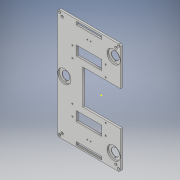
# Autodesk Inventor part: Grundplatte
Saved by Autodesk Inventor 2017 (Build 210142000, 142)
## iProperties
Part Number: Grundplatte
Material: Generisch
Document SubType Name: Modeling
Designer: Dima
Density: 1 g/cm^3
Appearance: Vorgabe
Author: Dima
Autodesk Inventor part; units mm, degrees
ref_plane "YZ Plane" through (0, 0, 0) normal (1, 0, 0) x (0, 1, 0)
ref_plane "XZ Plane" through (0, 0, 0) normal (0, 1, 0) x (-1, 0, 0)
ref_plane "XY Plane" through (0, 0, 0) normal (0, 0, 1) x (1, 0, 0)
sketch "Skizze1" plane through (0, 0, 0) normal (0, 1, 0) x (-1, 0, 0)
  line L0 (132.5635, 175.274) -> (-67.4365, 175.274)
  line L1 (-67.4365, 175.274) -> (-67.4365, -174.726)
  line L2 (-67.4365, -174.726) -> (132.5635, -174.726)
  line L3 (132.5635, -174.726) -> (132.5635, 175.274)
  line L4 (354.7243, 0.274) -> (-224.9528, 0.274)
  point P0 (0, 0)
  dimension "d0" = 350
  dimension "d1" = 200
  dimension "d2" = 175
  dimension "d3" = 175
  constraints: 10 end point, 2 horizontal, 2 parallel, 1 perpendicular
  measures "d0" distance of L2.end L0.start
  measures "d1" distance of L0.start L0.end
  measures "d2" distance between parallel lines of L0 L4
  measures "d3" distance between parallel lines of L2 L4
extrude "Extrusion1" add sketch "Skizze1" along normal blind 6
chamfer "Fase1" distance 5 angle 45 1 edges at (-132.5635, 3, 175.274)
chamfer "Fase2" distance 5 angle 45 1 edges at (67.4365, 3, 175.274)
chamfer "Fase3" distance 5 angle 45 1 edges at (67.4365, 3, -174.726)
chamfer "Fase4" distance 5 angle 45 1 edges at (-132.5635, 3, -174.726)
sketch "Skizze3" plane through (0, 6, 0) normal (0, 1, 0) x (1, 0, 0)
  point P0 (0, 0)
sketch "Skizze4" plane through (0, 6, 0) normal (0, 1, 0) x (1, 0, 0)
  point P0 (0, 0)
sketch "Skizze5" plane through (0, 6, 0) normal (0, 1, 0) x (1, 0, 0)
  line L0 (140.4629, -0.274) -> (-239.786, -0.274)
  line L1 (-32.5635, -205.6988) -> (-32.5635, 212.7513)
  line L2 (-127.5635, -175.274) -> (62.4365, -175.274) projected
  line L3 (62.4365, 174.726) -> (-127.5635, 174.726) projected
  line L4 (67.4365, -170.274) -> (67.4365, 169.726) projected
  line L5 (-132.5635, 169.726) -> (-132.5635, -170.274) projected
  line L6 (67.4365, -55.274) -> (-52.5635, -55.274)
  line L7 (-52.5635, -55.274) -> (-52.5635, 54.726)
  line L8 (-52.5635, 54.726) -> (67.4365, 54.726)
  line L9 (67.4365, 54.726) -> (67.4365, -55.274)
  point P0 (0, 0)
  dimension "d18" = 175
  dimension "d19" = 175
  dimension "d20" = 100
  dimension "d21" = 100
  dimension "d22" = 120
  dimension "d23" = 120
  dimension "d24" = 80
  dimension "d62" = 110
  constraints: 12 end point, 2 horizontal, 2 parallel, 1 perpendicular, 1 point on line, 1 vertical
  measures "d18" distance between parallel lines of L2 L0
  measures "d19" distance between parallel lines of L3 L0
  measures "d20" distance between parallel lines of L4 L1
  measures "d21" distance between parallel lines of L1 L5
  measures "d22" distance between parallel lines of L3 L8
  measures "d23" distance between parallel lines of L6 L2
  measures "d24" distance between parallel lines of L5 L7
  measures "d62" distance between parallel lines of L8 L6
extrude "Extrusion2" cut sketch "Skizze5" against normal blind 6
sketch "Skizze10" plane through (0, 6, 0) normal (0, 1, 0) x (1, 0, 0)
  line L0 (7.4365, -170.274) -> (-72.5635, -170.274)
  line L1 (-72.5635, -170.274) -> (-72.5635, -160.274)
  line L2 (-72.5635, -160.274) -> (7.4365, -160.274)
  line L3 (7.4365, -160.274) -> (7.4365, -170.274)
  line L4 (7.4365, 74.726) -> (-72.5635, 74.726)
  line L5 (-72.5635, 74.726) -> (-72.5635, 104.726)
  line L6 (-72.5635, 104.726) -> (7.4365, 104.726)
  line L7 (7.4365, 104.726) -> (7.4365, 74.726)
  line L8 (7.4365, 159.726) -> (-72.5635, 159.726)
  line L9 (-72.5635, 159.726) -> (-72.5635, 169.726)
  line L10 (-72.5635, 169.726) -> (7.4365, 169.726)
  line L11 (7.4365, 169.726) -> (7.4365, 159.726)
  line L12 (-52.5635, 54.726) -> (67.4365, 54.726) construction
  line L13 (67.4365, 54.726) -> (67.4365, 169.726) construction
  line L14 (62.4365, 174.726) -> (67.4365, 169.726) construction
  line L15 (62.4365, 174.726) -> (-127.5635, 174.726) construction
  line L16 (-132.5635, 169.726) -> (-127.5635, 174.726) construction
  line L17 (-132.5635, 169.726) -> (-132.5635, -170.274) construction
  line L18 (-127.5635, -175.274) -> (-132.5635, -170.274) construction
  line L19 (-127.5635, -175.274) -> (62.4365, -175.274) construction
  line L20 (67.4365, -170.274) -> (62.4365, -175.274) construction
  line L21 (67.4365, -170.274) -> (67.4365, -55.274) construction
  line L22 (67.4365, -55.274) -> (-52.5635, -55.274) construction
  line L23 (-52.5635, -55.274) -> (-52.5635, 54.726) construction
  line L24 (-127.5635, -175.274) -> (62.4365, -175.274) projected
  line L25 (7.4365, -105.274) -> (-72.5635, -105.274)
  line L26 (-72.5635, -105.274) -> (-72.5635, -75.274)
  line L27 (-72.5635, -75.274) -> (7.4365, -75.274)
  line L28 (7.4365, -75.274) -> (7.4365, -105.274)
  point P0 (0, 0)
  point P1 (-32.5635, -175.274)
  point P2 (-32.5635, -170.274)
  point P3 (-32.5635, -160.274)
  point P4 (-32.5635, 74.726)
  point P5 (-32.5635, -175.274)
  point P6 (-32.5635, 104.726)
  point P7 (-32.5635, 159.726)
  point P8 (-32.5635, -105.274)
  dimension "d99" = 5
  dimension "d100" = 10
  dimension "d101" = 10
  dimension "d102" = 5
  dimension "d106" = 55
  dimension "d107" = 55
  dimension "d108" = 30
  dimension "d109" = 30
  dimension "d110" = 80
  dimension "d111" = 80
  constraints: 32 end point, 8 midpoint, 8 parallel, 6 vertical alignment, 4 horizontal, 4 perpendicular
  measures "d99" distance between parallel lines of L0 L19
  measures "d100" distance between parallel lines of L2 L0
  measures "d101" distance between parallel lines of L10 L8
  measures "d102" distance between parallel lines of L15 L10
  measures "d106" distance between parallel lines of L2 L25
  measures "d107" distance between parallel lines of L8 L6
  measures "d108" distance between parallel lines of L25 L27
  measures "d109" distance of L4.end L5.end
  measures "d110" distance of L25.start L25.end
  measures "d111" distance of L0.start L0.end
extrude "Extrusion4" cut sketch "Skizze10" against normal through all
sketch "Skizze11" plane through (0, 0, 0) normal (0, -1, 0) x (1, 0, 0)
  line L0 (7.4365, -74.726) -> (7.4365, -104.726) construction
  line L1 (7.4365, -104.726) -> (-72.5635, -104.726) construction
  line L2 (-72.5635, -104.726) -> (-72.5635, -74.726) construction
  line L3 (-72.5635, -74.726) -> (7.4365, -74.726) construction
  line L4 (7.4365, 170.274) -> (7.4365, 160.274) construction
  line L5 (7.4365, 160.274) -> (-72.5635, 160.274) construction
  line L6 (-72.5635, 160.274) -> (-72.5635, 170.274) construction
  line L7 (-72.5635, 170.274) -> (7.4365, 170.274) construction
  line L8 (7.4365, -159.726) -> (7.4365, -169.726) construction
  line L9 (7.4365, -169.726) -> (-72.5635, -169.726) construction
  line L10 (-72.5635, -169.726) -> (-72.5635, -159.726) construction
  line L11 (-72.5635, -159.726) -> (7.4365, -159.726) construction
  line L12 (7.4365, 105.274) -> (7.4365, 75.274) construction
  line L13 (7.4365, 75.274) -> (-72.5635, 75.274) construction
  line L14 (-72.5635, 75.274) -> (-72.5635, 105.274) construction
  line L15 (-72.5635, 105.274) -> (7.4365, 105.274) construction
  line L16 (67.4365, -54.726) -> (-52.5635, -54.726) construction
  line L17 (-52.5635, -54.726) -> (-52.5635, 55.274) construction
  line L18 (-52.5635, 55.274) -> (67.4365, 55.274) construction
  line L19 (67.4365, 170.274) -> (67.4365, 55.274) construction
  line L20 (62.4365, 175.274) -> (67.4365, 170.274) construction
  line L21 (-127.5635, 175.274) -> (62.4365, 175.274) construction
  line L22 (-132.5635, 170.274) -> (-127.5635, 175.274) construction
  line L23 (-132.5635, -169.726) -> (-132.5635, 170.274) construction
  line L24 (-127.5635, -174.726) -> (-132.5635, -169.726) construction
  line L25 (62.4365, -174.726) -> (-127.5635, -174.726) construction
  line L26 (67.4365, -169.726) -> (62.4365, -174.726) construction
  line L27 (67.4365, -54.726) -> (67.4365, -169.726) construction
  circle A0 centre (-110.5635, 0.274) radius 21
  circle A1 centre (45.4365, 132.274) radius 21
  circle A2 centre (45.4365, -131.726) radius 21
  line L28 (-131.5635, -14.726) -> (-131.5635, 15.274) construction
  line L29 (-132.5635, -169.726) -> (-132.5635, 170.274) construction
  line L30 (66.4365, 132.274) -> (66.4365, 153.274) construction
  line L31 (66.4365, 153.274) -> (45.4365, 153.274) construction
  line L32 (45.4365, -152.726) -> (66.4365, -152.726) construction
  line L33 (66.4365, -152.726) -> (66.4365, -131.726) construction
  point P0 (0, 0)
  point P1 (-132.5635, 0.274)
  point P2 (-131.5635, 0.274)
  point P3 (-132.5635, 0.274)
  dimension "d114" = 42
  dimension "d115" = 42
  dimension "d116" = 42
  dimension "d117" = 30
  dimension "d118" = 1
  dimension "d119" = 1
  dimension "d120" = 22
  dimension "d121" = 22
  constraints: 10 end point, 5 tangent, 4 horizontal alignment, 3 centre point, 3 midpoint, 3 vertical alignment, 2 horizontal, 2 vertical, 1 perpendicular
  measures "d114" diameter of A0
  measures "d115" diameter of A1
  measures "d116" diameter of A2
  measures "d117" distance of L28.start L28.end
  measures "d118" distance between parallel lines of L23 L28
  measures "d119" distance between parallel lines of L19 L30
  measures "d120" distance between parallel lines of L25 L32
  measures "d121" distance between parallel lines of L21 L31
extrude "Extrusion5" cut sketch "Skizze11" against normal blind 5
sketch "Skizze12" plane through (45.4365, 5, -131.726) normal (0, -1, 0) x (1, 0, 0)
  circle A0 centre (0, 0) radius 21 projected
  circle A1 centre (-156, 132) radius 21 projected
  circle A2 centre (0, 264) radius 21 projected
  circle A3 centre (0, 264) radius 21 projected
  point P0 (-45.4365, 131.726)
  constraints: 3 coincident
hole "Bohrung1" at (-110.5635, 5, 0.274) at (45.4365, 5, 132.274) at (45.4365, 5, -131.726) direction (0, 1, 0) diameter 25 end through all
sketch "Skizze13" plane through (0, 0, 0) normal (0, -1, 0) x (1, 0, 0)
  circle A0 centre (45.4365, 132.274) radius 21 construction
  circle A1 centre (-110.5635, 0.274) radius 21 construction
  circle A2 centre (45.4365, -131.726) radius 21 construction
  line L0 (7.4365, -74.726) -> (7.4365, -104.726) construction
  line L1 (7.4365, -104.726) -> (-72.5635, -104.726) construction
  line L2 (-72.5635, -104.726) -> (-72.5635, -74.726) construction
  line L3 (-72.5635, -74.726) -> (7.4365, -74.726) construction
  line L4 (7.4365, 170.274) -> (7.4365, 160.274) construction
  line L5 (7.4365, 160.274) -> (-72.5635, 160.274) construction
  line L6 (-72.5635, 160.274) -> (-72.5635, 170.274) construction
  line L7 (-72.5635, 170.274) -> (7.4365, 170.274) construction
  line L8 (7.4365, -159.726) -> (7.4365, -169.726) construction
  line L9 (7.4365, -169.726) -> (-72.5635, -169.726) construction
  line L10 (-72.5635, -169.726) -> (-72.5635, -159.726) construction
  line L11 (-72.5635, -159.726) -> (7.4365, -159.726) construction
  line L12 (7.4365, 105.274) -> (7.4365, 75.274) construction
  line L13 (7.4365, 75.274) -> (-72.5635, 75.274) construction
  line L14 (-72.5635, 75.274) -> (-72.5635, 105.274) construction
  line L15 (-72.5635, 105.274) -> (7.4365, 105.274) construction
  line L16 (67.4365, -54.726) -> (-52.5635, -54.726) construction
  line L17 (-52.5635, -54.726) -> (-52.5635, 55.274) construction
  line L18 (-52.5635, 55.274) -> (67.4365, 55.274) construction
  line L19 (67.4365, 170.274) -> (67.4365, 55.274) construction
  line L20 (62.4365, 175.274) -> (67.4365, 170.274) construction
  line L21 (-127.5635, 175.274) -> (62.4365, 175.274) construction
  line L22 (-132.5635, 170.274) -> (-127.5635, 175.274) construction
  line L23 (-132.5635, -169.726) -> (-132.5635, 170.274) construction
  line L24 (-127.5635, -174.726) -> (-132.5635, -169.726) construction
  line L25 (62.4365, -174.726) -> (-127.5635, -174.726) construction
  line L26 (67.4365, -169.726) -> (62.4365, -174.726) construction
  line L27 (67.4365, -54.726) -> (67.4365, -169.726) construction
  point P0 (0, 0)
  point P1 (-125.5635, -167.726)
  point P2 (-117.5635, -159.726)
  point P3 (-125.5635, 168.274)
  point P4 (-117.5635, 160.274)
  point P5 (52.4365, 160.274)
  point P6 (60.4365, 168.274)
  point P7 (60.4365, -167.726)
  point P8 (52.4365, -159.726)
  dimension "d131" = 7
  dimension "d132" = 7
  dimension "d133" = 15
  dimension "d134" = 15
  dimension "d135" = 7
  dimension "d136" = 7
  dimension "d137" = 7
  dimension "d138" = 7
  dimension "d139" = 7
  dimension "d140" = 7
  dimension "d141" = 15
  dimension "d142" = 15
  dimension "d143" = 15
  dimension "d144" = 15
  dimension "d145" = 15
  dimension "d146" = 15
  measures "d131" distance from line of point (-125.564, -167.726) L25
  measures "d132" distance from line of L23 point (-125.564, -167.726)
  measures "d133" distance from line of L25 point (-117.564, -159.726)
  measures "d134" distance from line of L23 point (-117.564, -159.726)
  measures "d135" distance from line of L21 point (-125.564, 168.274)
  measures "d136" distance from line of L23 point (-125.564, 168.274)
  measures "d137" distance from line of L21 point (60.436, 168.274)
  measures "d138" distance from line of L19 point (60.436, 168.274)
  measures "d139" distance from line of L27 point (60.436, -167.726)
  measures "d140" distance from line of L25 point (60.436, -167.726)
  measures "d141" distance from line of L21 point (-117.564, 160.274)
  measures "d142" distance from line of L23 point (-117.564, 160.274)
  measures "d143" distance from line of L19 point (52.436, 160.274)
  measures "d144" distance from line of L21 point (52.436, 160.274)
  measures "d145" distance from line of L27 point (52.436, -159.726)
  measures "d146" distance from line of L25 point (52.436, -159.726)
hole "Bohrung2" at (60.4365, 0, -167.726) at (52.4365, 0, -159.726) at (-117.5635, 0, -159.726) at (-125.5635, 0, -167.726) at (-117.5635, 0, 160.274) at (-125.5635, 0, 168.274) at (52.4365, 0, 160.274) at (60.4365, 0, 168.274) direction (0, 1, 0) diameter 4.5 end through all counterbore diameter 8 counterbore depth 4
sketch "Skizze14" plane through (0, 0, 0) normal (0, -1, 0) x (1, 0, 0)
  circle A0 centre (52.4365, 160.274) radius 4 construction
  circle A1 centre (-117.5635, 160.274) radius 4 construction
  circle A2 centre (-117.5635, -159.726) radius 4 construction
  circle A3 centre (60.4365, -167.726) radius 4 construction
  circle A4 centre (52.4365, -159.726) radius 4 construction
  circle A5 centre (-125.5635, -167.726) radius 4 construction
  circle A6 centre (-125.5635, 168.274) radius 4 construction
  circle A7 centre (60.4365, 168.274) radius 4 construction
  circle A8 centre (45.4365, 132.274) radius 21 construction
  circle A9 centre (-110.5635, 0.274) radius 21 construction
  circle A10 centre (45.4365, -131.726) radius 21 construction
  line L0 (7.4365, -74.726) -> (7.4365, -104.726) construction
  line L1 (7.4365, -104.726) -> (-72.5635, -104.726) construction
  line L2 (-72.5635, -104.726) -> (-72.5635, -74.726) construction
  line L3 (-72.5635, -74.726) -> (7.4365, -74.726) construction
  line L4 (7.4365, 170.274) -> (7.4365, 160.274) construction
  line L5 (7.4365, 160.274) -> (-72.5635, 160.274) construction
  line L6 (-72.5635, 160.274) -> (-72.5635, 170.274) construction
  line L7 (-72.5635, 170.274) -> (7.4365, 170.274) construction
  line L8 (7.4365, -159.726) -> (7.4365, -169.726) construction
  line L9 (7.4365, -169.726) -> (-72.5635, -169.726) construction
  line L10 (-72.5635, -169.726) -> (-72.5635, -159.726) construction
  line L11 (-72.5635, -159.726) -> (7.4365, -159.726) construction
  line L12 (7.4365, 105.274) -> (7.4365, 75.274) construction
  line L13 (7.4365, 75.274) -> (-72.5635, 75.274) construction
  line L14 (-72.5635, 75.274) -> (-72.5635, 105.274) construction
  line L15 (-72.5635, 105.274) -> (7.4365, 105.274) construction
  line L16 (67.4365, -54.726) -> (-52.5635, -54.726) construction
  line L17 (-52.5635, -54.726) -> (-52.5635, 55.274) construction
  line L18 (-52.5635, 55.274) -> (67.4365, 55.274) construction
  line L19 (67.4365, 170.274) -> (67.4365, 55.274) construction
  line L20 (62.4365, 175.274) -> (67.4365, 170.274) construction
  line L21 (-127.5635, 175.274) -> (62.4365, 175.274) construction
  line L22 (-132.5635, 170.274) -> (-127.5635, 175.274) construction
  line L23 (-132.5635, -169.726) -> (-132.5635, 170.274) construction
  line L24 (-127.5635, -174.726) -> (-132.5635, -169.726) construction
  line L25 (62.4365, -174.726) -> (-127.5635, -174.726) construction
  line L26 (67.4365, -169.726) -> (62.4365, -174.726) construction
  line L27 (67.4365, -54.726) -> (67.4365, -169.726) construction
  line L28 (-32.5635, 105.274) -> (-32.5635, 75.274) construction
  point P0 (0, 0)
  point P1 (-85.0635, -97.226)
  point P2 (-85.0635, -62.226)
  point P3 (19.9365, -97.226)
  point P4 (19.9365, -62.226)
  point P5 (-85.0635, 62.774)
  point P6 (-85.0635, 97.774)
  point P7 (19.9365, 62.774)
  point P8 (19.9365, 97.774)
  dimension "d154" = 105
  dimension "d155" = 35
  dimension "d156" = 35
  dimension "d157" = 7.5
  dimension "d158" = 7.5
  constraints: 6 vertical alignment, 4 horizontal alignment, 2 end point, 2 midpoint, 1 symmetric about line
  measures "d154" distance of point (19.936, 97.774) point (-85.064, 97.774)
  measures "d155" distance of point (-85.064, 62.774) point (-85.064, 97.774)
  measures "d156" distance of point (-85.064, -97.226) point (-85.064, -62.226)
  measures "d157" distance from line of L18 point (19.936, 62.774)
  measures "d158" distance from line of L16 point (19.936, -62.226)
hole "Bohrung3" at (-85.0635, 0, -97.226) at (-85.0635, 0, -62.226) at (19.9365, 0, -97.226) at (19.9365, 0, -62.226) at (19.9365, 0, 62.774) at (19.9365, 0, 97.774) at (-85.0635, 0, 62.774) at (-85.0635, 0, 97.774) direction (0, 1, 0) diameter 4.134 depth 14.2 tip angle 118 thread size "M5x0.8" class "6H" standard "ISO Metric profile"
sketch "Skizze15" plane through (45.4365, 5, -131.726) normal (0, -1, 0) x (1, 0, 0)
  circle A0 centre (0, 264) radius 12.5 construction
  circle A1 centre (0, 0) radius 21 construction
  circle A2 centre (0, 0) radius 12.5 construction
  circle A3 centre (-156, 132) radius 21 construction
  circle A4 centre (-156, 132) radius 12.5 construction
  circle A5 centre (0, 264) radius 21 construction
  line L0 (0, -21) -> (0, 21) construction
  line L1 (-156, 111) -> (-156, 153) construction
  line L2 (0, 243) -> (0, 285) construction
  line L3 (-21, 264) -> (21, 264) construction
  line L4 (-177, 132) -> (-135, 132) construction
  line L5 (-178, -38) -> (-178, 302) construction
  line L6 (-21, 0) -> (21, 0) construction
  line L7 (22, 77) -> (22, -38) construction
  point P0 (-45.4365, 131.726)
  point P1 (0, 15)
  point P2 (0, -15)
  point P3 (-156, 117)
  point P4 (-156, 147)
  point P5 (0, 249)
  point P6 (0, 279)
  point P7 (0, 0)
  point P8 (0, 264)
  point P9 (-156, 132)
  dimension "d166" = 30
  dimension "d167" = 30
  dimension "d168" = 30
  constraints: 12 end point, 12 point on circle, 9 midpoint, 8 point on line, 3 symmetric about line, 2 perpendicular, 1 horizontal, 1 parallel, 1 vertical
  measures "d166" distance of point (-156, 147) point (-156, 117)
  measures "d167" distance of point (0, 15) point (0, -15)
  measures "d168" distance of point (0, 279) point (0, 249)
hole "Bohrung4" at (45.4365, 5, -146.726) at (45.4365, 5, -116.726) at (-110.5635, 5, -14.726) at (-110.5635, 5, 15.274) at (45.4365, 5, 117.274) at (45.4365, 5, 147.274) direction (0, 1, 0) diameter 2.459 depth 8.8 tip angle 118 thread size "M3x0.5" class "6H" standard "ISO Metric profile"
sketch "Skizze16" plane through (0, 0, 0) normal (0, -1, 0) x (1, 0, 0)
  circle A0 centre (-85.0635, 62.774) radius 2.067 construction
  circle A1 centre (19.9365, 62.774) radius 2.067 construction
  circle A2 centre (19.9365, -97.226) radius 2.067 construction
  circle A3 centre (-85.0635, -97.226) radius 2.067 construction
  circle A4 centre (-85.0635, -62.226) radius 2.067 construction
  circle A5 centre (19.9365, -62.226) radius 2.067 construction
  circle A6 centre (19.9365, 97.774) radius 2.067 construction
  circle A7 centre (-85.0635, 97.774) radius 2.067 construction
  circle A8 centre (52.4365, 160.274) radius 4 construction
  circle A9 centre (-117.5635, 160.274) radius 4 construction
  circle A10 centre (-117.5635, -159.726) radius 4 construction
  circle A11 centre (60.4365, -167.726) radius 4 construction
  circle A12 centre (52.4365, -159.726) radius 4 construction
  circle A13 centre (-125.5635, -167.726) radius 4 construction
  circle A14 centre (-125.5635, 168.274) radius 4 construction
  circle A15 centre (60.4365, 168.274) radius 4 construction
  circle A16 centre (45.4365, 132.274) radius 21 construction
  circle A17 centre (-110.5635, 0.274) radius 21 construction
  circle A18 centre (45.4365, -131.726) radius 21 construction
  line L0 (7.4365, -74.726) -> (7.4365, -104.726) construction
  line L1 (7.4365, -104.726) -> (-72.5635, -104.726) construction
  line L2 (-72.5635, -104.726) -> (-72.5635, -74.726) construction
  line L3 (-72.5635, -74.726) -> (7.4365, -74.726) construction
  line L4 (7.4365, 170.274) -> (7.4365, 160.274) construction
  line L5 (7.4365, 160.274) -> (-72.5635, 160.274) construction
  line L6 (-72.5635, 160.274) -> (-72.5635, 170.274) construction
  line L7 (-72.5635, 170.274) -> (7.4365, 170.274) construction
  line L8 (7.4365, -159.726) -> (7.4365, -169.726) construction
  line L9 (7.4365, -169.726) -> (-72.5635, -169.726) construction
  line L10 (-72.5635, -169.726) -> (-72.5635, -159.726) construction
  line L11 (-72.5635, -159.726) -> (7.4365, -159.726) construction
  line L12 (7.4365, 105.274) -> (7.4365, 75.274) construction
  line L13 (7.4365, 75.274) -> (-72.5635, 75.274) construction
  line L14 (-72.5635, 75.274) -> (-72.5635, 105.274) construction
  line L15 (-72.5635, 105.274) -> (7.4365, 105.274) construction
  line L16 (67.4365, -54.726) -> (-52.5635, -54.726) construction
  line L17 (-52.5635, -54.726) -> (-52.5635, 55.274) construction
  line L18 (-52.5635, 55.274) -> (67.4365, 55.274) construction
  line L19 (67.4365, 170.274) -> (67.4365, 55.274) construction
  line L20 (62.4365, 175.274) -> (67.4365, 170.274) construction
  line L21 (-127.5635, 175.274) -> (62.4365, 175.274) construction
  line L22 (-132.5635, 170.274) -> (-127.5635, 175.274) construction
  line L23 (-132.5635, -169.726) -> (-132.5635, 170.274) construction
  line L24 (-127.5635, -174.726) -> (-132.5635, -169.726) construction
  line L25 (62.4365, -174.726) -> (-127.5635, -174.726) construction
  line L26 (67.4365, -169.726) -> (62.4365, -174.726) construction
  line L27 (67.4365, -54.726) -> (67.4365, -169.726) construction
  line L28 (62.4365, -174.726) -> (-127.5635, -174.726) construction
  line L29 (-32.5635, -174.726) -> (-32.5635, 175.274) construction
  line L30 (-127.5635, 175.274) -> (62.4365, 175.274) construction
  point P0 (0, 0)
  point P1 (-37.5635, -136.726)
  point P2 (-27.5635, -136.726)
  point P3 (-37.5635, 137.274)
  point P4 (-27.5635, 137.274)
  dimension "d176" = 23
  dimension "d177" = 10
  dimension "d178" = 23
  constraints: 2 end point, 2 horizontal alignment, 2 midpoint, 2 vertical alignment, 1 symmetric about line
  measures "d176" distance from line of L11 point (-37.564, -136.726)
  measures "d177" distance of point (-37.564, -136.726) point (-27.564, -136.726)
  measures "d178" distance from line of point (-37.564, 137.274) L5
hole "Bohrung5" at (-37.5635, 0, -136.726) at (-27.5635, 0, -136.726) at (-37.5635, 0, 137.274) at (-27.5635, 0, 137.274) direction (0, 1, 0) diameter 3.242 depth 11.8 tip angle 118 thread size "M4x0.7" class "6H" standard "ISO Metric profile"
equation "\"d101\" = d100"
equation "\"d102\" = d99"
equation "\"d107\" = d106"
equation "\"d109\" = d108"
equation "\"d121\" = d120"
equation "\"d132\" = d131"
equation "\"d134\" = d133"
equation "\"d135\" = d131"
equation "\"d136\" = d131"
equation "\"d137\" = d131"
equation "\"d138\" = d131"
equation "\"d139\" = d131"
equation "\"d140\" = d131"
equation "\"d141\" = d133"
equation "\"d142\" = d133"
equation "\"d143\" = d133"
equation "\"d144\" = d133"
equation "\"d145\" = d133"
